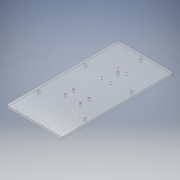
# Autodesk Inventor part: BT002_trajan20_21
Saved by Autodesk Inventor 2022.2 (Build 262287000, 287)
## iProperties
Company: HTBLA Kaindorf
RuleStatus: InUse
Created: 2022-08-03
Part Number: BT002_trajan20_21
Project: Zeichenmaschine_v2
Material: Acryl
Description: Platte Getriebemotor
Document SubType Name: Modeling
Designer: trajan20
Density: 1.188 g/cm^3
Appearance: Transparent - farblos
Mass: 169.723 g
Surface Area: 616.843 cm^2
Volume: 142.865 cm^3
AfterDocNew0: iProperties-Editor_aufrufen
Author: jan
Keywords: 2021
Autodesk Inventor part; units mm, degrees
ref_plane "YZ Plane" through (0, 0, 0) normal (1, 0, 0) x (0, 1, 0)
ref_plane "XZ Plane" through (0, 0, 0) normal (0, 1, 0) x (-1, 0, 0)
ref_plane "XY Plane" through (0, 0, 0) normal (0, 0, 1) x (1, 0, 0)
sketch "Skizze3" plane through (0, 0, 0) normal (0, 0, 1) x (1, 0, 0)
  line L0 (0, 0) -> (-120, 0)
  line L1 (-240, 0) -> (-240, 120)
  line L2 (-240, 120) -> (0, 120)
  line L3 (0, 120) -> (0, 0)
  line L4 (-248.2253, 60) -> (-229.9902, 60) construction
  line L5 (-189.05, 39.8483) -> (-189.05, 104.036) construction
  line L6 (-205.9145, 69.185) -> (-155.0384, 69.185) construction
  line L7 (-154.68, 50.3276) -> (-154.68, 100.4743) construction
  line L8 (-153.2541, 50.815) -> (-196.0103, 50.815) construction
  circle A0 centre (-180, 60) radius 3
  circle A1 centre (-189.05, 69.185) radius 1.35
  circle A2 centre (-189.05, 50.815) radius 1.35
  circle A3 centre (-154.68, 50.815) radius 1.35
  circle A4 centre (-154.68, 69.185) radius 1.35
  line L9 (-105, 40) -> (-80, 40)
  line L10 (-80, 40) -> (-80, 80)
  line L11 (-80, 80) -> (-105, 80)
  line L12 (-105, 80) -> (-105, 40)
  line L13 (-120, -37.5982) -> (-120, -22.8575) construction
  line L14 (-120, 0) -> (-240, 0)
  line L15 (-60, -24.367) -> (-60, 44.367) construction
  point P0 (-240, 60)
  point P1 (-105, 60)
  point P2 (-101.3, 43.7)
  point P3 (-230, 60)
  point P4 (-120, 120)
  point P5 (-180, 0)
  point P6 (-60, 0)
  point P7 (-60, 10)
  point P8 (-160, 10)
  point P9 (-160, 110)
  point P10 (-60, 110)
  point P11 (-60, 10)
  dimension "d4" = 120
  dimension "d5" = 240
  dimension "d6" = 60
  dimension "d8" = 9.05
  dimension "d9" = 34.37
  dimension "d11" = 9.185
  dimension "d12" = 18.37
  dimension "d13" = 2.7
  dimension "d14" = 2.7
  dimension "d15" = 2.7
  dimension "d16" = 2.7
  dimension "d17" = 6
  dimension "d18" = 40
  dimension "d19" = 25
  dimension "d20" = 75
  dimension "d21" = 3.7
  dimension "d22" = 3.7
  dimension "d39" = 10
  dimension "d40" = 10
  dimension "d41" = 10
  dimension "d42" = 10
  dimension "d43" = 10
  dimension "d51" = 80
  dimension "d52" = 80
  constraints: 32 end point, 16 point on line, 6 coincident, 6 horizontal, 6 midpoint, 5 centre point, 5 parallel, 4 vertical, 3 perpendicular
  measures "d4" distance between parallel lines of L0 L2
  measures "d5" distance between parallel lines of L1 L3
  measures "d6" distance from line of L1 point (-180, 60)
  measures "d8" distance from line of L5 point (-180, 60)
  measures "d9" distance between parallel lines of L5 L7
  measures "d11" distance from line of L6 point (-180, 60)
  measures "d12" distance between parallel lines of L8 L6
  measures "d13" diameter of A4
  measures "d14" diameter of A3
  measures "d15" diameter of A1
  measures "d16" diameter of A2
  measures "d17" diameter of A0
  measures "d18" distance between parallel lines of L11 L9
  measures "d19" distance between parallel lines of L12 L10
  measures "d20" distance from line of point (-180, 60) L12
  measures "d21" distance from line of L12 point (-101.3, 43.7)
  measures "d22" distance from line of L9 point (-101.3, 43.7)
  measures "d39" distance from line of L1 point (-230, 60)
  measures "d40" distance from line of L2 point (-60, 110)
  measures "d41" distance from line of L0 point (-60, 10)
  measures "d42" distance from line of L14 point (-160, 10)
  measures "d43" distance from line of L2 point (-160, 110)
  measures "d51" distance from line of L1 point (-160, 10)
  measures "d52" distance from line of L1 point (-160, 110)
extrude "Extrusion3" add sketch "Skizze3" against normal blind 5 contours L0 L14 L1 L2 L3 | L12 L11 L10 L9
hole "Bohrung1" at (-101.3, 43.7, 0) direction (0, 0, -1) diameter 4.134 end through all thread size "M5x0.8" class "6H" standard "ISO Metric profile"
pattern_linear "Rechteckige Anordnung1" count 2 spacing 32.6 along (0, 1, 0) count 2 spacing 17.6 along (1, 0, 0) of "Bohrung1"
fillet "Rundung1" radius 2 4 edges at (-240, 120, -2.5) (-240, 0, -2.5) (0, 120, -2.5) (0, 0, -2.5)
hole "Bohrung2" at (-230, 60, 0) at (-60, 10, 0) at (-160, 10, 0) at (-160, 110, 0) at (-60, 110, 0) direction (0, 0, -1) diameter 5.5 end through all
equation "\"d14\" = d13"
equation "\"d15\" = d13"
equation "\"d16\" = d15"
equation "\"d22\" = d21"
equation "\"d41\" = d40"
equation "\"d42\" = d41"
equation "\"d43\" = d42"
equation "\"d34\" = d18 - 2 * d22"
equation "\"d37\" = d19 - 2 * d21"
